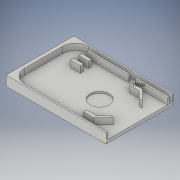
# Autodesk Inventor part: Playfield
Saved by Autodesk Inventor 2018 (Build 220112000, 112)
## iProperties
Created: 2018-10-08
Part Number: Playfield
Material: Generic
Document SubType Name: Modeling
Designer: zdaly3183
Density: 1 g/cm^3
Appearance: Default
Author: zdaly3183
Autodesk Inventor part; units mm, degrees
note: some values were not read from the file. Chosen so that the rebuilt part matches the saved one: direction of "Emboss1".
ref_plane "YZ Plane" through (0, 0, 0) normal (1, 0, 0) x (0, 1, 0)
ref_plane "XZ Plane" through (0, 0, 0) normal (0, 1, 0) x (-1, 0, 0)
ref_plane "XY Plane" through (0, 0, 0) normal (0, 0, 1) x (1, 0, 0)
sketch "Sketch1" plane through (0, 0, 0) normal (0, 1, 0) x (-1, 0, 0)
  line L0 (0, 0) -> (787.4, 0)
  line L1 (787.4, 0) -> (787.4, -533.4)
  line L2 (787.4, -533.4) -> (0, -533.4)
  line L3 (0, -533.4) -> (0, 0)
  dimension "d0" = 787.4
  dimension "d1" = 533.4
  constraints: 8 end point, 2 parallel, 1 horizontal, 1 perpendicular
  measures "d0" distance of L1.end L2.end
  measures "d1" distance of L0.end L1.end
extrude "Extrusion1" add sketch "Sketch1" along normal blind 25.4
sketch "Sketch2" plane through (0, 25.4, 0) normal (0, 1, 0) x (1, 0, 0)
  line L0 (-787.4, 0) -> (0, 0) projected
  line L1 (-787.4, 533.4) -> (-787.4, 0) projected
  line L2 (0, 0) -> (-787.4, 0)
  line L3 (-787.4, 0) -> (-787.4, 12.7)
  line L4 (-787.4, 12.7) -> (0, 12.7)
  line L5 (0, 12.7) -> (0, 0)
  line L6 (0, 533.4) -> (-787.4, 533.4) projected
  line L7 (0, 0) -> (0, 533.4) projected
  line L8 (-787.4, 533.4) -> (0, 533.4)
  line L9 (0, 533.4) -> (0, 520.7)
  line L10 (0, 520.7) -> (-787.4, 520.7)
  line L11 (-787.4, 520.7) -> (-787.4, 533.4)
  line L12 (-787.4, 533.4) -> (-762, 533.4)
  line L13 (-762, 533.4) -> (-762, 0)
  line L14 (-762, 0) -> (-787.4, 0)
  line L15 (-787.4, 0) -> (-787.4, 533.4)
  dimension "d4" = 12.7
  dimension "d5" = 12.7
  dimension "d6" = 25.4
  constraints: 24 end point, 6 parallel, 3 horizontal, 3 perpendicular, 3 point on line
  measures "d4" distance of L2.end L3.end
  measures "d5" distance of L8.end L9.end
  measures "d6" distance of L13.end L14.end
extrude "Extrusion2" add sketch "Sketch2" along normal blind 50.8 contours L1 L4 L13 L0 | L13 L4 L5 L0 | L1 L10 L13 L4 | L1 L6 L13 L10 | L13 L6 L7 L10
sketch "Sketch3" plane through (0, 25.4, 0) normal (0, 1, 0) x (1, 0, 0)
  line L0 (0, 533.4) -> (-787.4, 533.4) construction
  line L1 (0, 533.4) -> (0, 520.7) construction
  line L2 (0, 533.4) -> (0, 0) construction
  line L3 (0, 12.7) -> (0, 520.7) construction
  line L4 (0, 520.7) -> (0, 495.3) construction
  line L5 (-762, 520.7) -> (-762, 12.7) construction
  line L6 (-762, 520.7) -> (-762, 495.3) construction
  line L7 (0, 520.7) -> (-762, 520.7) construction
  line L8 (-762, 520.7) -> (-762, 419.1) construction
  line L9 (-762, 520.7) -> (-660.4, 520.7) construction
  arc A0 (-660.4, 520.7) -> (-762, 419.1) centre (-660.4, 419.1) ccw construction
  line L10 (0, 495.3) -> (-660.4, 495.3)
  line L11 (-660.4, 495.3) -> (-660.4, 482.6)
  line L12 (-660.4, 482.6) -> (0, 482.6)
  line L13 (0, 482.6) -> (0, 495.3)
  arc A1 (-660.4, 520.7) -> (-762, 419.1) centre (-660.4, 419.1) ccw
  line L14 (-762, 419.1) -> (-762, 520.7)
  line L15 (-762, 520.7) -> (-660.4, 520.7)
  dimension "d9" = 12.7
  dimension "d10" = 25.4
  dimension "d11" = 25.4
  dimension "d12" = 101.6
  dimension "d13" = 101.6
  dimension "d14" = 12.7
  constraints: 22 end point, 5 point on line, 4 point on circle, 2 centre point, 2 parallel, 2 tangent, 1 coincident, 1 collinear, 1 horizontal, 1 perpendicular
  measures "d9" distance of L0.start L1.end
  measures "d10" distance of L1.end L4.end
  measures "d11" distance of L5.start L6.end
  measures "d12" distance of L5.start L8.end
  measures "d13" distance of L5.start L9.end
  measures "d14" distance of L11.end L10.end
extrude "Extrusion3" add sketch "Sketch3" along normal blind 50.8
sketch "Sketch4" plane through (0, 25.4, 0) normal (0, 1, 0) x (1, 0, 0)
  line L0 (0, 12.7) -> (-762, 12.7) construction
  line L1 (-762, 12.7) -> (-654.2369, 120.4631) construction
  line L2 (-762, 12.7) -> (-609.6, 12.7) construction
  line L3 (-762, 419.1) -> (-762, 12.7) projected
  arc A0 (-762, 120.4631) -> (-654.2369, 12.7) centre (-654.2369, 120.4631) ccw
  line L4 (-654.2369, 12.7) -> (-762, 12.7)
  line L5 (-762, 120.4631) -> (-762, 12.7)
  point P0 (0, 0)
  dimension "d18" = 152.4
  dimension "d19" = 45
  constraints: 8 end point, 2 horizontal, 2 point on circle, 2 point on line, 1 centre point, 1 coincident, 1 equal length, 1 perpendicular, 1 tangent
  measures "d18" distance of L0.end L1.end
  measures "d19" angle of L2 L1
extrude "Extrusion4" add sketch "Sketch4" along normal blind 50.8
sketch "Sketch6" plane through (0, 76.2, 0) normal (0, 1, 0) x (1, 0, 0)
  line L0 (-660.4, 482.6) -> (0, 482.6) projected
  line L1 (-254.5688, 482.6) -> (-254.5688, 495.3)
  line L2 (0, 495.3) -> (-660.4, 495.3) projected
  line L3 (-254.5688, 482.6) -> (-305.3688, 482.6)
  line L4 (-305.3688, 482.6) -> (-305.3688, 495.3)
  line L5 (-305.3688, 495.3) -> (-254.5688, 495.3)
  point P0 (0, 0)
  dimension "d22" = 50.8
  constraints: 8 end point, 4 point on line, 1 collinear, 1 perpendicular, 1 vertical
  measures "d22" distance of L1.start L3.end
extrude "Extrusion5" cut sketch "Sketch6" against normal blind 50.8
sketch "Sketch8" plane through (0, 76.2, 0) normal (0, 1, 0) x (1, 0, 0)
  line L0 (-305.3688, 482.6) -> (-660.4, 482.6) projected
  line L1 (-660.4, 482.6) -> (-635, 482.6)
  line L2 (-635, 482.6) -> (-635, 495.3)
  line L3 (-305.3688, 495.3) -> (-660.4, 495.3) projected
  line L4 (-660.4, 495.3) -> (-635, 495.3)
  line L5 (-660.4, 482.6) -> (-660.4, 495.3) projected
  line L6 (-660.4, 482.6) -> (-660.4, 495.3)
  point P0 (0, 0)
  dimension "d26" = 25.4
  constraints: 8 end point, 2 collinear, 2 point on line, 1 perpendicular
  measures "d26" distance of L0.end L1.end
extrude "Extrusion6" cut sketch "Sketch8" against normal blind 50.8
sketch "Sketch7" plane through (0, 25.4, 0) normal (0, 1, 0) x (1, 0, 0)
  line L0 (-254.5688, 495.3) -> (-279.9688, 520.7) construction
  line L1 (0, 520.7) -> (-660.4, 520.7) construction
  line L2 (-254.5688, 495.3) -> (-218.6478, 495.3) construction
  point P0 (0, 0)
  dimension "d25" = 135
  constraints: 4 end point, 1 equal length, 1 horizontal, 1 point on line
  measures "d25" angle of L2 L0
sketch "Sketch9" plane through (0, 25.4, 0) normal (0, 1, 0) x (1, 0, 0)
  line L0 (0, 520.7) -> (-660.4, 520.7) construction
  line L1 (-635, 495.3) -> (-305.3688, 495.3) construction
  line L2 (-660.4, 520.7) -> (-635, 495.3) construction
  point P0 (0, 0)
  constraints: 2 end point
sketch "Sketch10" plane through (0, 25.4, 0) normal (0, 1, 0) x (1, 0, 0)
  line L0 (-635, 482.6) -> (-305.3688, 482.6) construction
  line L1 (-635, 482.6) -> (-635, 444.5) construction
  line L2 (-635, 444.5) -> (-635, 419.1) construction
  line L3 (-635, 419.1) -> (-635, 381) construction
  line L4 (-635, 381) -> (-635, 355.6) construction
  line L5 (-635, 355.6) -> (-558.8, 355.6)
  line L6 (-558.8, 355.6) -> (-558.8, 381)
  line L7 (-558.8, 381) -> (-635, 381)
  line L8 (-635, 381) -> (-635, 355.6)
  line L9 (-635, 419.1) -> (-558.8, 419.1)
  line L10 (-558.8, 419.1) -> (-558.8, 444.5)
  line L11 (-558.8, 444.5) -> (-635, 444.5)
  line L12 (-635, 444.5) -> (-635, 419.1)
  point P0 (0, 0)
  dimension "d29" = 38.1
  dimension "d30" = 25.4
  dimension "d31" = 38.1
  dimension "d32" = 25.4
  dimension "d33" = 76.2
  constraints: 24 end point, 4 parallel, 4 point on line, 2 horizontal, 2 perpendicular, 1 vertical
  measures "d29" distance of L0.start L1.end
  measures "d30" distance of L1.end L2.end
  measures "d31" distance of L2.end L3.end
  measures "d32" distance of L3.end L4.end
  measures "d33" distance of L7.end L6.end
extrude "Extrusion7" add sketch "Sketch10" along normal blind 50.8
sketch "Sketch11" plane through (0, 25.4, 0) normal (0, 1, 0) x (1, 0, 0)
  line L0 (0, 12.7) -> (0, 247.65) construction
  line L1 (0, 247.65) -> (-101.6, 247.65) construction
  line L2 (-101.6, 247.65) -> (-101.6, 209.55) construction
  line L3 (-101.6, 209.55) -> (-101.6, 133.35) construction
  line L4 (-101.6, 133.35) -> (-155.4815, 79.4685) construction
  line L5 (-155.4815, 79.4685) -> (-231.6815, 79.4685) construction
  line L6 (-101.6, 247.65) -> (-101.6, 361.95) construction
  line L7 (-101.6, 361.95) -> (-155.4815, 415.8315) construction
  line L8 (-155.4815, 415.8315) -> (-231.6815, 415.8315) construction
  line L9 (-155.4815, 79.4685) -> (-101.6, 133.35)
  line L10 (-101.6, 133.35) -> (-76.2, 133.35)
  line L11 (-76.2, 133.35) -> (-155.4815, 54.0685)
  line L12 (-155.4815, 54.0685) -> (-231.6815, 54.0685)
  line L13 (-231.6815, 54.0685) -> (-231.6815, 79.4685)
  line L14 (-231.6815, 79.4685) -> (-155.4815, 79.4685)
  line L15 (-101.6, 361.95) -> (-76.2, 361.95)
  line L16 (-76.2, 361.95) -> (-155.4815, 441.2315)
  line L17 (-155.4815, 441.2315) -> (-231.6815, 441.2315)
  line L18 (-231.6815, 441.2315) -> (-231.6815, 415.8315)
  line L19 (-155.4815, 415.8315) -> (-231.6815, 415.8315)
  line L20 (-155.4815, 415.8315) -> (-101.6, 361.95)
  point P0 (0, 0)
  dimension "d36" = 234.95
  dimension "d37" = 101.6
  dimension "d38" = 38.1
  dimension "d39" = 76.2
  dimension "d40" = 76.2
  dimension "d41" = 135
  dimension "d42" = 76.2
  dimension "d43" = 114.3
  dimension "d44" = 76.2
  dimension "d45" = 135
  dimension "d46" = 25.4
  constraints: 42 end point, 7 perpendicular, 4 collinear, 3 horizontal, 3 parallel, 2 vertical, 1 point on line
  measures "d36" distance of L0.start L0.end
  measures "d37" distance of L0.end L1.end
  measures "d38" distance of L1.end L2.end
  measures "d39" distance of L2.end L3.end
  measures "d40" distance of L3.end L4.end
  measures "d41" angle of L3 L4
  measures "d42" distance of L4.end L5.end
  measures "d43" distance of L1.end L6.end
  measures "d44" distance of L6.end L7.end
  measures "d45" angle of L7 L6
  measures "d46" distance of L3.end L10.end
extrude "Extrusion8" add sketch "Sketch11" along normal blind 50.8
sketch "Sketch12" plane through (0, 25.4, 0) normal (0, 1, 0) x (1, 0, 0)
  line L0 (0, 12.7) -> (0, 482.6) construction
  line L1 (0, 12.7) -> (0, 254) construction
  line L2 (0, 254) -> (-304.8, 254) construction
  circle A0 centre (-304.8, 254) radius 76.2
  point P0 (0, 0)
  dimension "d49" = 241.3
  dimension "d50" = 304.8
  dimension "d51" = 152.4
  constraints: 4 end point, 1 centre point, 1 coincident, 1 perpendicular, 1 point on line
  measures "d49" distance of L0.start L1.end
  measures "d50" distance of L1.end L2.end
  measures "d51" diameter of A0
emboss "Emboss1" sketch "Sketch12" operation cut depth 12.7 direction (0, -1, 0)
body "Solid1"
